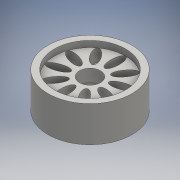
# Autodesk Inventor part: Wheel
Saved by Autodesk Inventor 2016 (Build 200138000, 138)
## iProperties
Created: 2016-12-01
Part Number: Wheel
Material: 一般
Document SubType Name: Modeling
Designer: KOTA-NPC2
Density: 1 g/cm^3
Appearance: 既定
Mass: 1.61263 g
Surface Area: 16.7191 cm^2
Volume: 1.61263 cm^3
Author: KOTA-NPC2
Autodesk Inventor part; units mm, degrees
ref_plane "YZ Plane" through (0, 0, 0) normal (1, 0, 0) x (0, 1, 0)
ref_plane "XZ Plane" through (0, 0, 0) normal (0, 1, 0) x (-1, 0, 0)
ref_plane "XY Plane" through (0, 0, 0) normal (0, 0, 1) x (1, 0, 0)
sketch "スケッチ1" plane through (0, 0, 0) normal (0, 0, 1) x (1, 0, 0)
  circle A0 centre (0, 0) radius 10
  circle A1 centre (0, 0) radius 5.8
  dimension "d0" = 20
  dimension "d1" = 11.6
  constraints: 2 centre point, 2 coincident
  measures "d0" diameter of A0
  measures "d1" diameter of A1
extrude "押し出し1" add sketch "スケッチ1" along normal blind 8.5 contours A0 | A1
extrude "押し出し2" cut sketch "スケッチ1" along normal blind 4 contours A1
sketch "スケッチ2" plane through (0, 0, 8.5) normal (0, 0, 1) x (1, 0, 0)
  circle A0 centre (0, 0) radius 6 construction
  ellipse E0 centre (0, 6) end of major axis (0, 3.5) minor radius 1
  ellipse E1 centre (-3.5267, 4.8541) end of major axis (-2.0572, 2.8316) minor radius 1
  circle A1 centre (0, 0) radius 6 construction
  ellipse E2 centre (-5.7063, 1.8541) end of major axis (-3.3287, 1.0816) minor radius 1
  circle A2 centre (0, 0) radius 6 construction
  ellipse E3 centre (-5.7063, -1.8541) end of major axis (-3.3287, -1.0816) minor radius 1
  circle A3 centre (0, 0) radius 6 construction
  ellipse E4 centre (-3.5267, -4.8541) end of major axis (-2.0572, -2.8316) minor radius 1
  circle A4 centre (0, 0) radius 6 construction
  ellipse E5 centre (0, -6) end of major axis (0, -3.5) minor radius 1
  circle A5 centre (0, 0) radius 6 construction
  ellipse E6 centre (3.5267, -4.8541) end of major axis (2.0572, -2.8316) minor radius 1
  circle A6 centre (0, 0) radius 6 construction
  ellipse E7 centre (5.7063, -1.8541) end of major axis (3.3287, -1.0816) minor radius 1
  circle A7 centre (0, 0) radius 6 construction
  ellipse E8 centre (5.7063, 1.8541) end of major axis (3.3287, 1.0816) minor radius 1
  circle A8 centre (0, 0) radius 6 construction
  ellipse E9 centre (3.5267, 4.8541) end of major axis (2.0572, 2.8316) minor radius 1
  circle A9 centre (0, 0) radius 6 construction
  circle A10 centre (0, 0) radius 2.5
  circle A11 centre (0, 0) radius 8.5
  dimension "d9" = 1
  dimension "d10" = 2.5
  dimension "d6" = 12
  dimension "d7" = 6
  dimension "d8" = 0
  dimension "d13" = 360
  dimension "d15" = 5
  dimension "d16" = 17
  constraints: 12 centre point, 5 coincident, 59 other
  measures "d6" diameter of A0
  measures "d7" distance of point (0, 0) point (0, 6)
  measures "d8" horizontal distance of point (0, 0) point (0, 6)
  measures "d15" diameter of A10
  measures "d16" diameter of A11
extrude "押し出し3" cut sketch "スケッチ2" against normal blind 4.5 contours E0 | E1 | E2 | E3 | E4 | E5 | E6 | E7 | E8 | E9 | A10
extrude "押し出し4" cut sketch "スケッチ2" against normal blind 1.5
sketch "表" plane through (0, 0, 8.5) normal (0, 0, 1) x (1, 0, 0)
  circle A0 centre (0, 0) radius 2.5 projected
  arc A1 (4.9962, 6.8766) -> (0, 8.5) centre (0, 0) ccw projected
  ellipse E0 centre (0, 6) end of major axis (0, 8.5) minor radius 1 projected
  arc A2 (0, 8.5) -> (-4.9962, 6.8766) centre (0, 0) ccw projected
  ellipse E1 centre (-3.5267, 4.8541) end of major axis (-4.9962, 6.8766) minor radius 1 projected
  arc A3 (-4.9962, 6.8766) -> (-8.084, 2.6266) centre (0, 0) ccw projected
  ellipse E2 centre (-5.7063, 1.8541) end of major axis (-8.084, 2.6266) minor radius 1 projected
  arc A4 (-8.084, 2.6266) -> (-8.084, -2.6266) centre (0, 0) ccw projected
  ellipse E3 centre (-5.7063, -1.8541) end of major axis (-8.084, -2.6266) minor radius 1 projected
  arc A5 (-8.084, -2.6266) -> (-4.9962, -6.8766) centre (0, 0) ccw projected
  ellipse E4 centre (-3.5267, -4.8541) end of major axis (-4.9962, -6.8766) minor radius 1 projected
  arc A6 (-4.9962, -6.8766) -> (0, -8.5) centre (0, 0) ccw projected
  ellipse E5 centre (0, -6) end of major axis (0, -8.5) minor radius 1 projected
  arc A7 (0, -8.5) -> (4.9962, -6.8766) centre (0, 0) ccw projected
  ellipse E6 centre (3.5267, -4.8541) end of major axis (4.9962, -6.8766) minor radius 1 projected
  arc A8 (4.9962, -6.8766) -> (8.084, -2.6266) centre (0, 0) ccw projected
  ellipse E7 centre (5.7063, -1.8541) end of major axis (8.084, -2.6266) minor radius 1 projected
  arc A9 (8.084, -2.6266) -> (8.084, 2.6266) centre (0, 0) ccw projected
  ellipse E8 centre (5.7063, 1.8541) end of major axis (8.084, 2.6266) minor radius 1 projected
  arc A10 (8.084, 2.6266) -> (4.9962, 6.8766) centre (0, 0) ccw projected
  ellipse E9 centre (3.5267, 4.8541) end of major axis (4.9962, 6.8766) minor radius 1 projected
  circle A11 centre (0, 0) radius 10 projected
  constraints: 2 vertical alignment, 8 other
sketch "裏" plane through (0, 0, 0) normal (0, 0, -1) x (-1, 0, 0)
  circle A0 centre (0, 0) radius 5.8 projected
  circle A1 centre (0, 0) radius 10 projected
